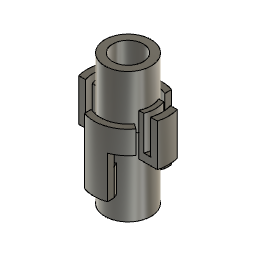
Connection v5 (Autodesk Fusion 360 design; units mm, degrees)
Autodesk Fusion 360 part; units mm, degrees
sketch "草图1" plane through (0, 0, 0) normal (0, 0, 1) x (1, 0, 0) in component "Component'"
  circle A0 centre (0, 0) radius 30
  dimension "d1" = 60
  constraint coincident A0.centre origin
  measures "d1" diameter of A0
extrude "拉伸1" add sketch "草图1" along normal blind 200 makes body 1 in component "Component'"
sketch "草图2" plane through (0, 0, 0) normal (0, 0, -1) x (1, 0, 0) in component "Component'"
  circle A0 centre (0, 0) radius 30
  circle A1 centre (0, 0) radius 53
  line L0 (-51.3809, 13) -> (51.3809, 13)
  line L1 (51.3809, -13) -> (-51.3809, -13)
  line L2 (1.75, 0) -> (22.5, 0)
  dimension "d4" = 106
  dimension "d5" = 26
  constraint concentric A0 A1
  constraint coincident A1 L0.start
  constraint coincident A1 L0.end
  constraint horizontal L0
  constraint coincident A1 L1.start
  constraint coincident A1 L1.end
  constraint parallel L0 L1
  constraint symmetric L0 L1 L2
  measures "d4" diameter of A1
  measures "d5" distance of L0 L1
extrude "拉伸2" add sketch "草图2" along normal blind 30 and the other way blind 25 contours A0 A1 L0 L1 | A0 A1 L0 L1 bodies 1 in component "Component'"
ref_plane "工作平面1" through (40.8536, 0, -20) normal (0, 0, -1) x (1, 0, 0) in component "Component'"
sketch "草图3" plane through (39.4089, 0, -20) normal (0, 0, -1) x (1, 0, 0) in component "Component'"
  circle A0 centre (-39.4089, 0) radius 30
  circle A1 centre (-39.4089, 0) radius 44.45
  circle A2 centre (-39.4089, 0) radius 36.1
  arc A3 (-90.7898, 13) -> (-90.7898, -13) centre (-39.4089, 0) ccw
  line L0 (-90.7898, 13) -> (-66.4459, 13)
  arc A4 (-66.4459, 13) -> (-66.4459, -13) centre (-39.4089, 0) ccw
  line L1 (-66.4459, -13) -> (-90.7898, -13)
  arc A5 (11.972, -13) -> (11.972, 13) centre (-39.4089, 0) ccw
  line L2 (11.972, -13) -> (-12.3719, -13)
  arc A6 (-12.3719, -13) -> (-12.3719, 13) centre (-39.4089, 0) ccw
  line L3 (-12.3719, 13) -> (11.972, 13)
  line L4 (-12.3719, 13) -> (11.972, 13)
  point P0 (3.0508, 13)
  point P1 (-5.7309, 13)
  point P2 (3.0976, -13)
  point P3 (-5.7309, -13)
  point P4 (-73.0869, 13)
  point P5 (-81.9154, 13)
  point P6 (-73.0869, -13)
  point P7 (-81.9154, -13)
  dimension "d11" = 88.9
  dimension "d12" = 72.2
  constraint concentric A0 A1
  constraint concentric A1 A2
  constraint coincident L3 P0
  constraint coincident L3 P1
  constraint coincident A2 P1
  constraint coincident L2 P2
  constraint coincident A1 P2
  constraint coincident L2 P3
  constraint coincident A2 P3
  constraint coincident A2 P4
  constraint coincident L0 P4
  constraint coincident A1 P5
  constraint coincident L0 P5
  constraint coincident A2 P6
  constraint coincident L1 P6
  constraint coincident A1 P7
  constraint coincident L1 P7
  measures "d11" diameter of A1
  measures "d12" diameter of A2
sketch "草图4" plane through (0, 0, -30) normal (0, 0, -1) x (1, 0, 0) in component "Component'"
  arc A0 (-51.3809, 13) -> (-51.3809, -13) centre (0, 0) ccw
  line L0 (-51.3809, -13) -> (-27.037, -13)
  arc A1 (-27.037, 13) -> (-27.037, -13) centre (0, 0) ccw
  line L1 (-27.037, 13) -> (-51.3809, 13)
  circle A2 centre (0, 0) radius 44.45
  circle A3 centre (0, 0) radius 36.1
  line L2 (-51.3809, 13) -> (-27.037, 13)
  line L3 (-27.037, -13) -> (-51.3809, -13)
  line L4 (27.037, 13) -> (51.3809, 13)
  line L5 (51.3809, -13) -> (27.037, -13)
extrude "拉伸3" cut sketch "草图4" against normal blind 45 contours L0 L1 A2 A3 L2 L3 | A2 A3 L4 L5 bodies 1 in component "Component'"
extrude "拉伸4" add sketch "草图3" along normal blind 10 contours A1 A2 L2 L3 L4 | A1 A2 L0 L1 bodies 1 in component "Component'"
sketch "草图1 (2)" plane through (0, 0, 0) normal (0, 0, -1) x (1, 0, 0) in component "Component''"
  arc A0 (-27.037, 13) -> (-27.037, -13) centre (0, 0) ccw
  arc A1 (-27.037, -13) -> (27.037, -13) centre (0, 0) ccw
  arc A2 (27.037, -13) -> (27.037, 13) centre (0, 0) ccw
  arc A3 (27.037, 13) -> (-27.037, 13) centre (0, 0) ccw
  circle A4 centre (0, 0) radius 30
  constraint coincident A0.centre A1.centre
extrude "拉伸1'" add sketch "草图1 (2)" along normal blind 400 separate body makes body 2 in component "Component''"
ref_plane "工作平面2" through (0, 0, -45) normal (0, 0, -1) x (-1, 0, 0) in component "Component''"
sketch "草图4 (2)" plane through (0, 0, -45) normal (0, 0, -1) x (1, 0, 0) in component "Component''"
  circle A0 centre (0, 0) radius 36.27
  circle A1 centre (0, 0) radius 44.41
  line L0 (15, 41.8001) -> (15, -41.8001)
  line L1 (-15, -41.8001) -> (-15, 41.8001)
  line L2 (0, -1.75) -> (0, -22.5)
  dimension "d21" = 72.54
  dimension "d22" = 88.82
  dimension "d23" = 30
  constraint coincident A0.centre A1.centre
  constraint coincident A1 L0.start
  constraint coincident A1 L0.end
  constraint vertical L0
  constraint coincident A1 L1.start
  constraint coincident A1 L1.end
  constraint parallel L0 L1
  constraint symmetric L0 L1 L2
  measures "d21" diameter of A0
  measures "d22" diameter of A1
  measures "d23" distance of L0 L1
extrude "拉伸2'" add sketch "草图4 (2)" against normal blind 60 separate body contours A0 A1 L0 L1 | A0 A1 L0 L1 makes body 3 at (13.4193, 33.6962, -5) makes body 4 at (-11.8085, -34.2939, -25) in component "Component''"
sketch "草图5" plane through (0, 0, -45) normal (0, 0, -1) x (1, 0, 0) in component "Component''"
  arc A0 (-15, -41.8001) -> (15, -41.8001) centre (0, 0) ccw
  line L0 (15, -41.8001) -> (15, -33.0229)
  arc A1 (-15, -33.0229) -> (15, -33.0229) centre (0, 0) ccw
  line L1 (-15, -33.0229) -> (-15, -41.8001)
  arc A2 (15, 41.8001) -> (-15, 41.8001) centre (0, 0) ccw
  line L2 (-15, 41.8001) -> (-15, 33.0229)
  arc A3 (15, 33.0229) -> (-15, 33.0229) centre (0, 0) ccw
  line L3 (15, 33.0229) -> (15, 41.8001)
  circle A4 centre (0, 0) radius 36.27
  circle A5 centre (0, 0) radius 30
  dimension "d26" = 72.54
  constraint coincident A0.centre A1.centre
  measures "d26" diameter of A4
extrude "拉伸3'" add sketch "草图5" against normal blind 10 contours A1 A3 A4 bodies 2 3 4 in component "Component''"
extrude "拉伸4'" add 1 faces at (10.2577, -35.2464, -45) along direction (0, 0, -1) blind 10 on bodies 2 bodies 2 in component "Component''"
sketch "草图6" plane through (0, 0, 15) normal (0, 0, 1) x (-1, 0, 0) in component "Component''"
  arc A0 (-15, -41.8001) -> (15, -41.8001) centre (0, 0) ccw
  line L0 (15, -41.8001) -> (15, -33.0229)
  arc A1 (-15, -33.0229) -> (15, -33.0229) centre (0, 0) ccw
  line L1 (-15, -33.0229) -> (-15, -41.8001)
  circle A2 centre (0, 0) radius 36.27
  circle A3 centre (0, 0) radius 44.41
  line L2 (0, 0) -> (36.1229, -25.8338)
  line L3 (0, 0) -> (15, -33.0229)
  line L4 (0, 0) -> (-15, 33.0229)
  line L5 (0, 0) -> (-29.5018, 21.0987)
  line L6 (-29.5018, 21.0987) -> (-36.1229, 25.8338)
  line L7 (-15, 33.0229) -> (-15, 41.8001)
  line L8 (15, -33.0229) -> (15, -41.8001)
  dimension "d31" = 72.54
  dimension "d32" = 88.82
  dimension "d33" = 30
  dimension "d34" = 30
  constraint coincident A0.centre A1.centre
  constraint coincident A3 L2.end
  constraint coincident L0.end A1.end
  constraint coincident A2 L4.end
  constraint parallel L3 L4
  constraint coincident A2 L5.end
  constraint coincident A3 L6.end
  constraint parallel L5 L6
  constraint coincident A3 L7.end
  constraint vertical L7
  constraint coincident A0.end L0.start
  measures "d31" diameter of A2
  measures "d32" diameter of A3
  measures "d33" angle of L2 L3
  measures "d34" angle of L4 L5
extrude "拉伸5" add sketch "草图6" against normal blind 30 contours L0 A2 A3 L2 L8 | A2 A3 L6 L7 bodies 2 in component "Component''"
sketch "草图5 (2)" plane through (0, 0, 200) normal (0, 0, 1) x (-1, 0, 0) in component "Component'"
  circle A0 centre (0, 0) radius 30
  circle A1 centre (0, 0) radius 20
  dimension "d37" = 40
  constraint coincident A0.centre A1.centre
  measures "d37" diameter of A1
extrude "拉伸5'" cut sketch "草图5 (2)" against normal through all contours A1 bodies 1 in component "Component'"
extrude "拉伸6" cut sketch "草图5 (2)" against normal through all contours A1 bodies 2 in component "Component''"
extrude "拉伸6'" cut 1 faces at (26.4805, -2.484, 200) along direction (0, 0, -1) blind 130 on bodies 1 bodies 1 in component "Component'"
extrude "拉伸7" cut 1 faces at (-24.9403, -9.2401, -400) along direction (0, 0, 1) blind 300 on bodies 2 bodies 2 in component "Component''"
sketch "草图1 (3)" plane through (0, 0, 25) normal (0, 0, 1) x (-1, 0, 0)
  arc A0 (51.3809, -13) -> (51.3809, 13) centre (0, 0) ccw
  line L0 (51.3809, 13) -> (27.037, 13)
  arc A1 (27.037, -13) -> (27.037, 13) centre (0, 0) ccw
  line L1 (27.037, -13) -> (51.3809, -13)
  arc A2 (42.5065, -13) -> (42.5065, 13) centre (0, 0) ccw
  line L2 (42.5065, -13) -> (33.678, -13)
  arc A3 (33.678, -13) -> (33.678, 13) centre (0, 0) ccw
  line L3 (33.678, 13) -> (42.5065, 13)
  line L4 (-33.678, -13) -> (-42.5065, -13)
  arc A4 (-42.5065, 13) -> (-42.5065, -13) centre (0, 0) ccw
  line L5 (-42.5065, 13) -> (-33.678, 13)
  arc A5 (-33.678, 13) -> (-33.678, -13) centre (0, 0) ccw
extrude "拉伸7'" cut sketch "草图1 (3)" against normal blind 10 contours L0 L1 A2 L2 A3 L3 | L4 A4 L5 A5 bodies 1 in component "Component'"
sketch "草图7" plane through (0, 0, -35) normal (0, 0, 1) x (-1, 0, 0) in component "Component''"
  circle A0 centre (0, 0) radius 30
  arc A1 (15, -33.0229) -> (15, 33.0229) centre (0, 0) ccw
  arc A2 (15, 33.0229) -> (-15, 33.0229) centre (0, 0) ccw
  arc A3 (-15, 33.0229) -> (-15, -33.0229) centre (0, 0) ccw
  arc A4 (-15, -33.0229) -> (15, -33.0229) centre (0, 0) ccw
  arc A5 (-15, -41.8001) -> (36.1229, -25.8338) centre (0, 0) ccw
  line L0 (36.1229, -25.8338) -> (29.5018, -21.0987)
  arc A6 (-15, -33.0229) -> (29.5018, -21.0987) centre (0, 0) ccw
  line L1 (-15, -33.0229) -> (-15, -41.8001)
  arc A7 (15, 41.8001) -> (-36.1229, 25.8338) centre (0, 0) ccw
  line L2 (-36.1229, 25.8338) -> (-29.5018, 21.0987)
  arc A8 (15, 33.0229) -> (-29.5018, 21.0987) centre (0, 0) ccw
  line L3 (15, 33.0229) -> (15, 41.8001)
  line L4 (0, 0) -> (29.5018, -21.0987)
  line L5 (0, 0) -> (-15, -33.0229)
  line L6 (-29.5018, 21.0987) -> (0, 0)
  circle A9 centre (0, 0) radius 20
  circle A10 centre (0, 0) radius 30
  line L7 (0, 0) -> (15, 33.0229)
  line L8 (-15, 33.0229) -> (0, 0)
  line L9 (0, 0) -> (15, -33.0229)
  point P0 (12.4069, 27.3142)
  point P1 (24.4019, -17.4514)
  point P2 (-12.4069, -27.3142)
  point P3 (-24.4019, 17.4514)
  constraint coincident A0.centre A1.centre
  constraint coincident L0.end A6.end
  constraint coincident A3.end A4.start
  constraint coincident L2.end A8.end
  constraint coincident A10 P0
  constraint coincident L4 P1
  constraint coincident A10 P1
  constraint coincident L5 P2
  constraint coincident A0 P2
  constraint coincident L6 P3
  constraint coincident A0 P3
  constraint coincident A1.end A2.start
  constraint coincident A2.end A3.start
  constraint coincident A1.start A4.end
extrude "拉伸8" cut sketch "草图7" against normal blind 20 contours A0 A1 L4 A10 L7 | A0 A1 A6 L4 A10 L9 | A0 A3 A8 L6 A10 L8 | A0 A3 L5 L6 A10 bodies 2 in component "Component''"
extrude "拉伸9" add 2 faces at (10.8428, -35.0945, -55) (10.8428, 35.0945, -55) along direction (0, 0, -1) blind 15 on bodies 2 bodies 2 in component "Component''"
component "Component'" placed x (1, 0, 0) y (0, 1, 0) z (0, 0, 1) at (0, 0, 0)
component "Component''" placed x (1, 0, 0) y (0, 1, 0) z (0, 0, 1) at (0, 0, 0)
